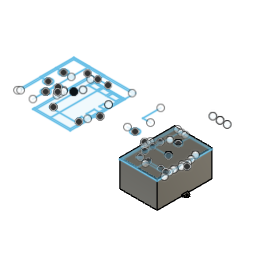
Trab-RICA2 v16 (Autodesk Fusion 360 design; units mm, degrees)
Autodesk Fusion 360 part; units mm, degrees
sketch "Esboço1" plane through (0, 0, 0) normal (0, 0, 1) x (1, 0, 0)
  line L0 (-57.5, 57.5) -> (62.5, 57.5)
  line L1 (62.5, 57.5) -> (62.5, -52.5)
  line L2 (-57.5, -52.5) -> (-57.5, 57.5)
  line L3 (-54.5, -49.5) -> (-54.5, 54.5)
  line L4 (-54.5, 54.5) -> (59.5, 54.5)
  line L5 (-57.5, 57.5) -> (2.5, 57.5)
  line L6 (2.5, 54.5) -> (2.5, 44.5)
  circle A0 centre (2.5, 44.5) radius 3
  line L7 (2.5, 44.5) -> (22.5, 44.5)
  line L8 (2.5, 44.5) -> (-17.5, 44.5)
  circle A1 centre (-17.5, 44.5) radius 3
  circle A2 centre (22.5, 44.5) radius 3
  line L9 (-57.5, 57.5) -> (-27.5, 57.5)
  line L10 (-27.5, 57.5) -> (-27.5, -52.5)
  line L11 (-57.5, 57.5) -> (-57.5, 22.5)
  line L12 (-57.5, 22.5) -> (-42.5, 22.5)
  circle A3 centre (-42.5, 22.5) radius 7.5
  line L13 (-57.5, 22.5) -> (-57.5, -7.5)
  line L14 (-57.5, -7.5) -> (-42.5, -7.5)
  circle A4 centre (-42.5, -7.5) radius 7.5
  line L15 (-27.5, -7.5) -> (-12.5, -7.5)
  circle A5 centre (-27.5, 22.5) radius 3.5
  line L16 (-27.5, -7.5) -> (-27.5, -27.5)
  circle A6 centre (-27.5, -27.5) radius 7.5
  line L17 (-25.25, -25.75) -> (-29.75, -25.75)
  line L18 (-29.75, -25.75) -> (-29.75, -29.25)
  line L19 (-29.75, -29.25) -> (-25.25, -29.25)
  line L20 (-25.25, -29.25) -> (-25.25, -25.75)
  line L21 (-29.4343, -26.0657) -> (-29.4343, -28.9343)
  line L22 (-29.4343, -28.9343) -> (-25.5657, -28.9343)
  line L23 (-25.5657, -28.9343) -> (-25.5657, -26.0657)
  line L24 (-25.5657, -26.0657) -> (-29.4343, -26.0657)
  line L25 (59.5, 35.5) -> (2.5, 35.5)
  line L26 (2.5, 35.5) -> (2.5, -49.5)
  line L27 (59.5, -49.5) -> (56, -49.5)
  line L28 (56, -49.5) -> (56, -46)
  line L29 (2.5, -49.5) -> (6, -49.5)
  line L30 (6, -49.5) -> (6, -46)
  circle A7 centre (6, 12) radius 1.375
  circle A8 centre (6, 12) radius 3
  circle A9 centre (6, -46) radius 1.375
  circle A10 centre (6, -46) radius 3
  circle A11 centre (56, -46) radius 1.375
  circle A12 centre (56, -46) radius 3
  circle A13 centre (56, 12) radius 1.375
  circle A14 centre (56, 12) radius 3
  line L31 (59.5, -49.5) -> (59.5, -38.9)
  line L32 (59.5, -38.9) -> (59.5, -42.9)
  line L33 (59.5, -38.9) -> (59.5, -34.9)
  line L34 (59.5, -42.9) -> (56, -42.9)
  line L35 (59.5, -49.5) -> (59.5, -17.5)
  line L36 (59.5, -17.5) -> (59.5, -25)
  line L37 (59.5, -25) -> (59.5, -32.5)
  line L38 (59.5, -17.5) -> (59.5, -10)
  line L39 (59.5, -49.5) -> (59.5, 4)
  line L40 (59.5, 4) -> (59.5, 0)
  line L41 (59.5, 4) -> (59.5, 8)
  line L42 (59.5, 35.5) -> (49.25, 35.5)
  line L43 (49.25, 35.5) -> (57.25, 35.5)
  line L44 (49.25, 35.5) -> (41.25, 35.5)
  line L45 (41.25, 35.5) -> (41.25, 25)
  line L46 (57.25, 35.5) -> (57.25, 25)
  line L47 (59.5, 35.5) -> (30.5, 35.5)
  line L48 (30.5, 35.5) -> (38, 35.5)
  line L49 (30.5, 35.5) -> (23, 35.5)
  line L50 (38, 35.5) -> (38, 25)
  line L51 (38, 25) -> (23, 25)
  line L52 (41.25, 25) -> (57.25, 25)
  line L53 (59.5, 35.5) -> (12.5, 35.5)
  line L54 (12.5, 35.5) -> (20, 35.5)
  line L55 (12.5, 35.5) -> (5, 35.5)
  line L56 (23, 35.5) -> (23, 25)
  line L57 (20, 35.5) -> (20, 25)
  line L58 (20, 25) -> (5, 25)
  line L59 (5, 25) -> (5, 35.5)
  line L60 (59.5, 8) -> (50, 8)
  line L61 (50, 8) -> (50, 0)
  line L62 (59.5, 0) -> (50, 0)
  line L63 (59.5, -10) -> (50, -10)
  line L64 (50, -10) -> (50, -25)
  line L65 (50, -25) -> (59.5, -25)
  line L66 (59.5, -34.9) -> (50, -34.9)
  line L67 (50, -34.9) -> (50, -42.9)
  line L68 (56, -42.9) -> (50, -42.9)
  line L69 (59.5, 37.5) -> (2.5, 37.5)
  line L70 (2.5, 37.5) -> (-7.5, 37.5)
  line L71 (59.5, 37.5) -> (62.5, 37.5)
  circle A15 centre (-23.226, -7.5) radius 6.5
  line L72 (-7.5, 37.5) -> (-4.5, 37.5)
  line L73 (2.5, 35.5) -> (-7.5, 35.5)
  line L74 (2.5, -49.5) -> (59.5, -49.5)
  line L75 (62.5, -52.5) -> (62.5, -55.5)
  line L76 (59.5, -52.5) -> (59.5, -49.5)
  line L77 (-10.5, -66.5) -> (-10.5, 37.5)
  line L78 (-10.5, 37.5) -> (-7.5, 37.5)
  line L79 (-7.5, -66.5) -> (-7.5, 35.5)
  line L80 (59.5, 35.5) -> (59.5, 8)
  line L81 (21.2759, 35.5) -> (21.2759, -66.5)
  line L82 (21.2759, -66.5) -> (-10.5, -66.5)
  line L83 (-10.5, -66.5) -> (-10.5, -69.5)
  line L84 (-10.5, -69.5) -> (62.5, -69.5)
  line L85 (62.5, -69.5) -> (62.5, -55.5)
  line L86 (21.2759, -66.5) -> (59.5, -66.5)
  line L87 (59.5, -66.5) -> (59.5, -52.5)
  line L88 (62.5, 37.5) -> (62.5, -16)
  line L89 (62.5, -16) -> (67.5, -16)
  circle A16 centre (67.5, -16) radius 1.5
  circle A17 centre (67.5, -16) radius 4
  line L90 (62.5, -22.3696) -> (69.0157, -19.7017)
  line L91 (69.0783, -12.3245) -> (62.5, -9.4998)
  line L92 (-17.0783, -19.675) -> (-10.5, -22.4998)
  circle A18 centre (-15.5, -15.9996) radius 1.5
  line L93 (-10.5, -9.6299) -> (-17.0157, -12.2978)
  circle A19 centre (-15.5, -15.9996) radius 4
  line L94 (-10.5, -15.9996) -> (-15.5, -15.9996)
  point P0 (-27.5, -27.5)
  dimension "d1" = 120
  dimension "d2" = 110
  dimension "d4" = 10
  dimension "d5" = 6
  dimension "d6" = 20
  dimension "d7" = 20
  dimension "d8" = 6
  dimension "d9" = 6
  dimension "d10" = 30
  dimension "d11" = 35
  dimension "d12" = 15
  dimension "d13" = 15
  dimension "d14" = 30
  dimension "d15" = 15
  dimension "d16" = 15
  dimension "d19" = 15
  dimension "d20" = 7
  dimension "d22" = 20
  dimension "d23" = 15
  dimension "d24" = 4.5
  dimension "d25" = 3.5
  dimension "d26" = -0.3157
  dimension "d57" = 57
  dimension "d58" = 57
  dimension "d59" = 3.5
  dimension "d60" = 3.5
  dimension "d61" = 3.5
  dimension "d62" = 3.5
  dimension "d63" = 58
  dimension "d64" = 58
  dimension "d65" = 2.75
  dimension "d66" = 6
  dimension "d67" = 2.75
  dimension "d68" = 6
  dimension "d69" = 2.75
  dimension "d70" = 6
  dimension "d71" = 2.75
  dimension "d72" = 6
  dimension "d73" = 10.6
  dimension "d74" = 4
  dimension "d75" = 4
  dimension "d76" = 32
  dimension "d77" = 7.5
  dimension "d79" = 7.5
  dimension "d80" = 53.5
  dimension "d81" = 4
  dimension "d82" = 4
  dimension "d83" = 10.25
  dimension "d84" = 8
  dimension "d85" = 8
  dimension "d86" = 29
  dimension "d87" = 7.5
  dimension "d88" = 7.5
  dimension "d89" = 47
  dimension "d90" = 7.5
  dimension "d91" = 7.5
  dimension "d92" = 2
  dimension "d94" = 13
  dimension "d95" = 3
  dimension "d118" = 3
  dimension "d131" = 102
  dimension "d132" = 3
  dimension "d242" = 53.5
  dimension "d243" = 5
  dimension "d244" = 3
  dimension "d245" = 8
  dimension "d246" = 5
  dimension "d247" = 3
  dimension "d248" = 8
  constraint horizontal L0
  constraint perpendicular L0 L1
  constraint parallel L1 L2
  constraint midpoint L0 L5.end
  constraint midpoint L4 L6.start
  constraint perpendicular L4 L6
  constraint coincident L6.end A0.centre
  constraint perpendicular L6 L7
  constraint coincident L8.end A1.centre
  constraint coincident L7.end A2.centre
  constraint perpendicular L2 L9
  constraint perpendicular L9 L11
  constraint perpendicular L3 L12
  constraint coincident L12.end A3.centre
  constraint perpendicular L12 L13
  constraint perpendicular L13 L14
  constraint coincident L14.end A4.centre
  constraint coincident L10 L15.start
  constraint perpendicular L10 L15
  constraint perpendicular L15 L16
  constraint coincident P0 L16.end
  constraint horizontal L17
  constraint perpendicular L17 L18
  constraint parallel L17 L19
  constraint parallel L18 L20
  constraint perpendicular L26 L29
  constraint perpendicular L29 L30
  constraint concentric A7 A8
  constraint coincident L30.end A9.centre
  constraint concentric A9 A10
  constraint coincident L28.end A11.centre
  constraint concentric A13 A14
  constraint perpendicular L27 L31
  constraint parallel L31 L32
  constraint perpendicular L27 L35
  constraint parallel L35 L36
  constraint parallel L35 L37
  constraint parallel L39 L40
  constraint parallel L42 L43
  constraint parallel L25 L44
  constraint perpendicular L25 L45
  constraint perpendicular L43 L46
  constraint parallel L25 L47
  constraint parallel L47 L48
  constraint parallel L25 L49
  constraint perpendicular L25 L50
  constraint perpendicular L50 L51
  constraint perpendicular L46 L52
  constraint parallel L25 L53
  constraint parallel L25 L54
  constraint parallel L25 L55
  constraint perpendicular L51 L56
  constraint perpendicular L53 L57
  constraint perpendicular L57 L58
  constraint perpendicular L25 L59
  constraint perpendicular L41 L60
  constraint perpendicular L60 L61
  constraint perpendicular L61 L62
  constraint perpendicular L39 L63
  constraint perpendicular L63 L64
  constraint perpendicular L39 L66
  constraint perpendicular L34 L67
  constraint perpendicular L67 L68
  constraint coincident L1 L71.end
  constraint perpendicular L1 L71
  constraint coincident L15 A15.centre
  constraint perpendicular L26 L74
  constraint parallel L1 L75
  constraint perpendicular L27 L76
  constraint perpendicular L73 L79
  constraint perpendicular L60 L80
  constraint coincident L25 L81.start
  constraint coincident L79.start L82
  constraint perpendicular L79 L82
  constraint perpendicular L77 L82
  constraint perpendicular L82 L83
  constraint perpendicular L75 L84
  constraint perpendicular L84 L85
  constraint perpendicular L76 L86
  constraint perpendicular L71 L88
  constraint perpendicular L1 L89
  constraint coincident L89.end A16.centre
  constraint concentric A16 A17
  constraint coincident L1 L90.start
  constraint coincident A17 L90.end
  constraint tangent A17 L90
  constraint coincident A17 L91.start
  constraint coincident L1 L91.end
  constraint tangent A17 L91
  constraint coincident A18.centre A19.centre
  constraint concentric A18 A19
  constraint coincident L93.end A19
  constraint tangent L93 A19
  constraint coincident L92.start A19
  constraint tangent L92 A19
  measures "d1" distance of L1.end L2.start
  measures "d2" distance of L0.end L1.end
  measures "d4" distance of L6.start L6.end
  measures "d5" diameter of A0
  measures "d6" distance of L6.end L7.end
  measures "d7" distance of L6.end L8.end
  measures "d8" diameter of A1
  measures "d9" diameter of A2
  measures "d10" distance of L0.start L9.end
  measures "d11" distance of L0.start L11.end
  measures "d12" distance of L11.end L12.end
  measures "d13" diameter of A3
  measures "d14" distance of L11.end L13.end
  measures "d15" distance of L13.end L14.end
  measures "d16" diameter of A4
  measures "d19" distance of L15.start L15.end
  measures "d20" diameter of A5
  measures "d22" distance of L15.start P0
  measures "d23" diameter of A6
  measures "d24" distance of L18.end L19.end
  measures "d25" distance of L17.end L18.end
  measures "d57" distance of L27.start L26.end
  measures "d58" distance of L25.start L25.end
  measures "d59" distance of L27.start L27.end
  measures "d60" distance of L27.end L28.end
  measures "d61" distance of L26.end L29.end
  measures "d62" distance of L29.end L30.end
  measures "d63" distance of L30.end A7.centre
  measures "d64" distance of L28.end A13.centre
  measures "d65" diameter of A7
  measures "d66" diameter of A8
  measures "d67" diameter of A9
  measures "d68" diameter of A10
  measures "d69" diameter of A11
  measures "d70" diameter of A12
  measures "d71" diameter of A13
  measures "d72" diameter of A14
  measures "d73" distance of L27.start L31.end
  measures "d74" distance of L31.end L32.end
  measures "d75" distance of L31.end L33.end
  measures "d76" distance of L27.start L35.end
  measures "d77" distance of L35.end L36.end
  measures "d79" distance of L35.end L38.end
  measures "d80" distance of L27.start L39.end
  measures "d81" distance of L39.end L40.end
  measures "d82" distance of L39.end L41.end
  measures "d83" distance of L25.start L42.end
  measures "d84" distance of L42.end L43.end
  measures "d85" distance of L42.end L44.end
  measures "d86" distance of L25.start L47.end
  measures "d87" distance of L47.end L48.end
  measures "d88" distance of L47.end L49.end
  measures "d89" distance of L25.start L53.end
  measures "d90" distance of L53.end L54.end
  measures "d91" distance of L53.end L55.end
  measures "d94" diameter of A15
  measures "d95" distance of L70.end L72.end
  measures "d118" distance of L1.end L75.end
  measures "d131" distance of L81.start L81.end
  measures "d132" distance of L77.start L83.end
  measures "d242" distance of L71.end L88.end
  measures "d243" distance of L88.end L89.end
  measures "d244" diameter of A16
  measures "d245" diameter of A17
  measures "d246" distance of L94.start A18.centre
  measures "d247" diameter of A18
  measures "d248" diameter of A19
sketch "Esboço2" plane through (0, 0, 0) normal (0, 0, 1) x (1, 0, 0)
  line L0 (121.4343, 17.9343) -> (117.5657, 17.9343)
  circle A0 centre (119.5, 16.5) radius 7.5
  line L1 (92.5, 57.5) -> (152.5, 57.5)
  circle A1 centre (121.5, 44.5) radius 3
  line L2 (209.5, 54.5) -> (209.5, -49.5)
  line L3 (117.5657, 17.9343) -> (117.5657, 15.0657)
  line L4 (121.4343, 15.0657) -> (121.4343, 17.9343)
  circle A2 centre (113.3812, 29.2702) radius 3.5
  line L5 (212.5, 57.5) -> (212.5, -52.5)
  line L6 (121.5, 44.5) -> (107.5, 44.5)
  line L7 (92.5, 57.5) -> (122.5, 57.5)
  line L8 (98.3812, 29.2702) -> (113.3812, 29.2702)
  line L9 (209.5, -49.5) -> (95.5, -49.5)
  line L10 (92.5, -7.5) -> (107.5, -7.5)
  line L11 (121.75, 14.75) -> (121.75, 18.25)
  line L12 (121.5, 44.5) -> (135.5, 44.5)
  line L13 (121.75, 18.25) -> (117.25, 18.25)
  circle A3 centre (107.5, 44.5) radius 3
  line L14 (117.25, 14.75) -> (121.75, 14.75)
  circle A4 centre (127.764, 29.9834) radius 5
  line L15 (92.5, 22.5) -> (107.5, 22.5)
  line L16 (95.5, 54.5) -> (209.5, 54.5)
  line L17 (92.5, -52.5) -> (92.5, 57.5)
  line L18 (117.5657, 15.0657) -> (121.4343, 15.0657)
  line L19 (95.5, -49.5) -> (95.5, 54.5)
  line L20 (212.5, -52.5) -> (92.5, -52.5)
  line L21 (92.5, 57.5) -> (212.5, 57.5)
  circle A5 centre (135.5, 44.5) radius 3
  line L22 (117.25, 18.25) -> (117.25, 14.75)
  line L23 (92.5, 57.5) -> (92.5, 22.5)
  line L24 (92.5, 22.5) -> (92.5, -7.5)
  line L25 (95.5, 6.594) -> (145, 6.594)
  line L26 (145, 6.594) -> (145, 54.5)
  point P0 (150, 0)
  point P1 (150, 0)
  point P2 (119.5, 16.5)
  dimension "d29" = 3
  dimension "d30" = -0.3157
  dimension "d31" = 120
  dimension "d32" = 110
  dimension "d34" = 6
  dimension "d37" = 6
  dimension "d38" = 6
  dimension "d39" = 30
  dimension "d40" = 35
  dimension "d43" = 30
  dimension "d46" = 15
  dimension "d48" = 7
  dimension "d49" = 10
  dimension "d51" = 15
  dimension "d52" = 4.5
  dimension "d53" = 3.5
  constraint horizontal L21
  constraint perpendicular L5 L21
  constraint parallel L20 L21
  constraint parallel L5 L17
  constraint coincident P1 P0
  constraint midpoint L1.end L21
  constraint coincident A1.centre L6.start
  constraint coincident L6.end A3.centre
  constraint coincident L12.end A5.centre
  constraint perpendicular L7 L17
  constraint perpendicular L7 L23
  constraint perpendicular L15 L19
  constraint perpendicular L15 L24
  constraint perpendicular L10 L24
  constraint coincident A2.centre L8.end
  constraint horizontal L13
  constraint perpendicular L13 L22
  constraint parallel L13 L14
  constraint parallel L11 L22
  constraint coincident L19 L25.start
  constraint perpendicular L19 L25
  constraint coincident L16 L26.end
  constraint perpendicular L16 L26
  measures "d31" distance of L17.start L5.end
  measures "d32" distance of L5.start L5.end
  measures "d34" diameter of A1
  measures "d37" diameter of A3
  measures "d38" diameter of A5
  measures "d39" distance of L1.start L7.end
  measures "d40" distance of L1.start L15.start
  measures "d43" distance of L15.start L10.start
  measures "d46" distance of L8.start A2.centre
  measures "d48" diameter of A2
  measures "d49" diameter of A4
  measures "d51" diameter of A0
  measures "d52" distance of L11.start L14.start
  measures "d53" distance of L13.end L14.start
extrude "Extrusão2" add sketch "Esboço2" along normal blind 3 contours A0 | L16 L19 L25 L26 | L11 L13 L14 L22 makes body 1
extrude "Extrusão3" add sketch "Esboço1" along normal blind 30 separate body contours L1 L69 L70 L71 L72 L75 L77 L78 L83 L84 L85 L88 makes body 2
extrude "Extrusão4" add sketch "Esboço1" along normal blind 3 contours L25 L27 L31 L34 L35 L37 L39 L42 L45 L46 L47 L50 L51 L52 L53 L56 L60 L61 L62 L63 L64 L65 L66 L67 L68 L74 L80 L81 | L25 L42 L43 L44 L45 L46 L47 L52 L53 | L39 L40 L41 L60 L61 L62 | L25 L47 L48 L49 L50 L51 L53 L56 | L35 L36 L38 L39 L63 L64 L65 | L25 L26 L29 L53 L57 L58 L59 L74 L81 | L25 L53 L54 L55 L57 L58 L59 | L26 L29 L73 L74 L79 L81 L82 | L27 L74 L76 L81 L86 L87 | L31 L32 L33 L34 L35 L39 L66 L67 L68 | A7 | A8 | A13 | A14 bodies 2
extrude "Extrusão6" add sketch "Esboço1" along normal blind 8 contours A8 | A10 | A12 | A14 bodies 2
sketch "Esboço3" plane through (0, 37.5, 0) normal (0, 1, 0) x (-1, 0, 0)
  line L0 (-62.5, 0) -> (10.5, 0)
  line L1 (10.5, 30) -> (-62.5, 30)
  line L2 (-62.5, 30) -> (-62.5, 0)
  line L3 (-59.5623, 0) -> (-59.5623, 8)
  line L4 (-2.4095, 0) -> (-2.4095, 8)
  line L5 (-59.5623, 8) -> (-2.4095, 8)
  line L6 (-59.5623, 8) -> (-59.5623, 23)
  line L7 (-2.4095, 8) -> (-2.4095, 23)
  line L8 (-59.5623, 23) -> (-2.4095, 23)
  line L9 (10.5, 0) -> (10.5, 30)
  dimension "d104" = 8
  dimension "d105" = 8
  dimension "d106" = 15
  dimension "d107" = 15
  constraint coincident L0 L3.start
  constraint perpendicular L0 L3
  constraint coincident L0 L4.start
  constraint perpendicular L0 L4
  constraint perpendicular L5 L6
  constraint perpendicular L5 L7
  constraint perpendicular L7 L8
  measures "d104" distance of L3.start L3.end
  measures "d105" distance of L4.start L4.end
  measures "d106" distance of L3.end L6.end
  measures "d107" distance of L4.end L7.end
extrude "Extrusão7" cut sketch "Esboço3" against normal blind 5 contours L5 L6 L7 L8 bodies 2
sketch "Esboço4" plane through (62.5, 0, 0) normal (1, 0, 0) x (0, 1, 0)
  line L0 (-69.5, 0) -> (37.5, 0)
  line L1 (37.5, 0) -> (37.5, 30)
  line L2 (37.5, 30) -> (-69.5, 30)
  line L3 (-43.5, 0) -> (-43.5, 8)
  line L4 (9, 0) -> (9, 8)
  line L5 (-43.5, 8) -> (9, 8)
  line L6 (-43.5, 8) -> (-43.5, 16)
  line L7 (-43.5, 16) -> (9, 16)
  line L8 (9, 16) -> (9, 8)
  line L9 (-69.5, 30) -> (-69.5, 0)
  dimension "d111" = 8
  dimension "d112" = 8
  dimension "d113" = 8
  constraint coincident L0 L3.start
  constraint perpendicular L0 L3
  constraint coincident L0 L4.start
  constraint perpendicular L0 L4
  constraint perpendicular L4 L5
  constraint perpendicular L5 L6
  constraint perpendicular L4 L7
  constraint perpendicular L5 L8
  measures "d111" distance of L3.start L3.end
  measures "d112" distance of L4.start L4.end
  measures "d113" distance of L3.end L6.end
extrude "Extrusão8" cut sketch "Esboço4" against normal blind 5 contours L5 L6 L7 L8 bodies 2
sketch "Esboço5" plane through (0, 0, 3) normal (0, 0, 1) x (-1, 0, 0)
  line L0 (-59.5, -35.5) -> (7.5, -35.5)
  line L1 (-1.5, 53.5) -> (-1.5, 65.5)
  line L2 (7.5, -35.5) -> (7.5, -34.5)
  line L3 (7.5, -34.5) -> (-1.5, -34.5)
  line L4 (-1.5, -34.5) -> (-1.5, -22.5)
  line L5 (7.5, -22.5) -> (7.5, -34.5)
  line L6 (7.5, -35.5) -> (7.5, 66.5)
  line L7 (-1.5, 53.5) -> (7.5, 53.5)
  line L8 (-1.5, 65.5) -> (7.5, 65.5)
  line L9 (7.5, 65.5) -> (7.5, 53.5)
  line L10 (7.5, -22.5) -> (-1.5, -22.5)
  line L11 (7.5, 65.5) -> (4.5, 65.5)
  line L12 (4.5, 65.5) -> (4.5, -34.5)
  line L13 (7.5, -34.5) -> (7.5, 65.5)
  line L14 (7.5, 66.5) -> (-59.5, 66.5)
  circle A0 centre (-56, -12) radius 3
  line L15 (-59.5, 66.5) -> (-59.5, -35.5)
  circle A1 centre (-56, 46) radius 3
  circle A2 centre (-6, 46) radius 3
  circle A3 centre (-6, -12) radius 3
  line L16 (-56.5, 53.5) -> (-47.5, 53.5)
  line L17 (-47.5, 65.5) -> (-50.5, 65.5)
  line L18 (-56.5, 65.5) -> (-47.5, 65.5)
  line L19 (-56.5, 53.5) -> (-56.5, 65.5)
  line L20 (-47.5, 65.5) -> (-47.5, 53.5)
  line L21 (-56.5, 65.5) -> (-53.5, 65.5)
  line L22 (-53.5, 65.5) -> (-53.5, 53.5)
  line L23 (4.5, -22.5) -> (-1.5, -34.5)
  line L24 (-1.5, -22.5) -> (4.5, -34.5)
  circle A4 centre (1.5, -28.5) radius 1.25
  line L25 (-1.5, 53.5) -> (4.5, 65.5)
  line L26 (4.5, 53.5) -> (-1.5, 65.5)
  circle A5 centre (1.5, 59.5) radius 1.25
  line L27 (-53.5, 53.5) -> (-47.5, 65.5)
  line L28 (-47.5, 53.5) -> (-53.5, 65.5)
  circle A6 centre (-50.5, 59.5) radius 1.25
  dimension "d117" = 12
  dimension "d120" = 1
  dimension "d121" = 9
  dimension "d122" = 12
  dimension "d126" = 9
  dimension "d127" = 9
  dimension "d128" = 3
  dimension "d133" = 12
  dimension "d134" = 9
  dimension "d135" = 9
  dimension "d137" = 3
  dimension "d148" = 2.5
  dimension "d232" = 2.5
  dimension "d233" = 2.5
  constraint coincident L0.end L2.start
  constraint perpendicular L0 L2
  constraint perpendicular L3 L4
  constraint perpendicular L1 L7
  constraint perpendicular L6 L8
  constraint perpendicular L7 L9
  constraint perpendicular L4 L10
  constraint perpendicular L6 L11
  constraint coincident L3 L12.end
  constraint perpendicular L3 L12
  constraint perpendicular L8 L13
  constraint perpendicular L16 L19
  constraint perpendicular L16 L20
  constraint perpendicular L19 L21
  constraint coincident L16 L22.end
  constraint perpendicular L16 L22
  constraint coincident L12 L23.start
  constraint coincident L10 L23.start
  constraint midpoint L24 A4.centre
  constraint coincident L7 L26.start
  constraint coincident L12 L26.start
  constraint midpoint L25 A5.centre
  constraint midpoint L27 A6.centre
  measures "d117" distance of L1.start L1.end
  measures "d120" distance of L0.end L2.end
  measures "d121" distance of L2.end L3.end
  measures "d122" distance of L3.end L4.end
  measures "d126" distance of L1.start L7.end
  measures "d127" distance of L1.end L8.end
  measures "d128" distance of L8.end L11.end
  measures "d133" distance of L18.start L16.start
  measures "d134" distance of L16.start L16.end
  measures "d135" distance of L18.start L17.start
  measures "d137" distance of L18.start L21.end
  measures "d148" diameter of A4
  measures "d232" diameter of A5
  measures "d233" diameter of A6
extrude "Extrusão9" add sketch "Esboço5" along normal blind 37 separate body contours L3 L5 L6 L10 L12 L13 | L6 L7 L8 L9 L11 L12 L13 | L16 L18 L19 L21 L22 makes body 3 at (-7.5, -57.5, 27.6667) makes body 4 at (-7.5, 26.5, 15.3333) makes body 5 at (56.5, -57.5, 27.6667)
sketch "Esboço6" plane through (0, 0, 40) normal (0, 0, 1) x (-1, 0, 0)
  line L0 (7.5, 53.5) -> (7.5, 65.5)
  line L1 (7.5, 65.5) -> (4.5, 65.5)
  line L2 (4.5, 65.5) -> (4.5, 53.5)
  line L3 (4.5, -34.5) -> (7.5, -34.5)
  line L4 (7.5, 65.5) -> (-56.5, 65.5)
  line L5 (-56.5, 65.5) -> (-56.5, 53.5)
  line L6 (4.5, 53.5) -> (7.5, 53.5)
  line L7 (7.5, -34.5) -> (7.5, -22.5)
  line L8 (7.5, -22.5) -> (4.5, -22.5)
  line L9 (4.5, -22.5) -> (4.5, -34.5)
  line L10 (7.5, 65.5) -> (7.5, -34.5)
  line L11 (7.5, -34.5) -> (-56.5, -34.5)
  line L12 (-56.5, -34.5) -> (-56.5, 65.5)
  line L13 (4.5, 62.5) -> (-53.5, 62.5)
  line L14 (-53.5, -31.5) -> (-53.5, 62.5)
  line L15 (4.5, -31.5) -> (-53.5, -31.5)
  line L16 (4.5, 62.5) -> (4.5, -31.5)
  dimension "d147" = 3
  constraint coincident L0.end L1.start
  constraint perpendicular L0 L4
  constraint perpendicular L3 L5
  constraint coincident L3.end L7.start
  constraint perpendicular L5 L11
  constraint perpendicular L4 L12
hole "Furo1" at (50.5, -59.5, 3) direction (0, 0, -1) diameter 2.5 depth 2 tip angle 118 bodies 2
hole "Furo2" at (-1.5, 28.5, 3) at (-1.5, -59.5, 3) direction (0, 0, -1) diameter 2.5 depth 2 tip angle 118 bodies 2
extrude "Extrusão11" add sketch "Esboço6" along normal blind 2 contours L0 L1 L2 L4 L6 L10 L16 | L6 L8 L10 L16 | L3 L7 L8 L9 L10 L11 L16 | L2 L4 L5 L9 L11 L12 L13 L14 L15 bodies 2 5 3 4
sketch "Esboço7" plane through (0, 0, 0) normal (0, 0, 1) x (1, 0, 0)
  line L0 (229.5, 35.5) -> (172.5, 35.5)
  line L1 (182.5, 35.5) -> (175, 35.5)
  line L2 (172.5, 35.5) -> (172.5, -49.5)
  line L3 (172.5, 35.5) -> (162.5, 35.5)
  line L4 (172.5, 37.5) -> (162.5, 37.5)
  line L5 (229.5, 37.5) -> (172.5, 37.5)
  line L6 (112.5, 57.5) -> (112.5, 22.5)
  line L7 (112.5, 22.5) -> (127.5, 22.5)
  line L8 (112.5, -7.5) -> (127.5, -7.5)
  circle A0 centre (127.5, -7.5) radius 7.5
  line L9 (159.5, -66.5) -> (159.5, 37.5)
  line L10 (162.5, -66.5) -> (162.5, 35.5)
  line L11 (159.5, -69.5) -> (232.5, -69.5)
  line L12 (172.5, -49.5) -> (229.5, -49.5)
  line L13 (229.5, 4) -> (229.5, 0)
  line L14 (229.5, -49.5) -> (229.5, 4)
  line L15 (229.5, 35.5) -> (229.5, 8)
  circle A1 centre (226, 12) radius 3
  circle A2 centre (226, 12) radius 1.375
  line L16 (229.5, 4) -> (229.5, 8)
  circle A3 centre (226, -46) radius 3
  circle A4 centre (226, -46) radius 1.375
  line L17 (229.5, -49.5) -> (226, -49.5)
  line L18 (226, -49.5) -> (226, -46)
  line L19 (229.5, -52.5) -> (229.5, -49.5)
  line L20 (229.5, -66.5) -> (229.5, -52.5)
  line L21 (229.5, -49.5) -> (229.5, -38.9)
  line L22 (229.5, -49.5) -> (229.5, -17.5)
  circle A5 centre (176, 12) radius 3
  circle A6 centre (176, 12) radius 1.375
  circle A7 centre (176, -46) radius 3
  circle A8 centre (176, -46) radius 1.375
  line L23 (176, -49.5) -> (176, -46)
  line L24 (172.5, -49.5) -> (176, -49.5)
  line L25 (229.5, -38.9) -> (229.5, -42.9)
  line L26 (229.5, -38.9) -> (229.5, -34.9)
  line L27 (159.5, -69.5) -> (159.5, -66.5)
  line L28 (162.5, -66.5) -> (229.5, -66.5)
  line L29 (232.5, -52.5) -> (232.5, -69.5)
  line L30 (159.5, 37.5) -> (162.5, 37.5)
  line L31 (229.5, 37.5) -> (232.5, 37.5)
  line L32 (232.5, -52.5) -> (232.5, 37.5)
  line L33 (159.5, -69.5) -> (159.5, -16)
  line L34 (159.5, -16) -> (170, -16)
  circle A9 centre (205.5, 94.5) radius 3
  circle A10 centre (191.5, 94.5) radius 3
  circle A11 centre (177.5, 94.5) radius 3
  circle A12 centre (191.5, 94.5) radius 3
  circle A13 centre (205.5, 94.5) radius 3
  circle A14 centre (177.5, 94.5) radius 3
  circle A15 centre (191.5, 94.5) radius 3
  circle A16 centre (170, -16) radius 3.25
  line L35 (170, -16) -> (170, -31)
  circle A17 centre (170, -31) radius 3.25
  line L36 (170, -16) -> (170, -1)
  circle A18 centre (170, -1) radius 3.25
  line L37 (162.5, -66.5) -> (190.5, -66.5)
  line L38 (190.5, -66.5) -> (190.5, -45)
  line L39 (190.5, 35.5) -> (190.5, 14)
  circle A19 centre (190.5, -45) radius 3.5
  circle A20 centre (190.5, 14) radius 6
  line L40 (173.25, -16.0046) -> (201.25, -16.0046)
  line L41 (190.5, -45) -> (215.5, -45)
  circle A21 centre (215.5, -45) radius 5
  line L42 (199.5, -13.7546) -> (203, -13.7546)
  line L43 (203, -13.7546) -> (203, -18.2546)
  line L44 (203, -18.2546) -> (199.5, -18.2546)
  line L45 (199.5, -18.2546) -> (199.5, -13.7546)
  line L46 (199.5, -13.7546) -> (203, -18.2546) construction
  line L47 (203, -13.7546) -> (199.5, -18.2546) construction
  line L48 (199.81, -17.9446) -> (199.81, -14.0646)
  line L49 (199.81, -14.0646) -> (202.69, -14.0646)
  line L50 (202.69, -14.0646) -> (202.69, -17.9446)
  line L51 (202.69, -17.9446) -> (199.81, -17.9446)
  circle A22 centre (201.25, -16.0046) radius 5
  line L52 (239.0783, -12.3245) -> (232.5, -9.4998)
  circle A23 centre (237.5, -16) radius 1.5
  line L53 (232.5, -22.3696) -> (239.0157, -19.7017)
  circle A24 centre (237.5, -16) radius 4
  line L54 (232.5, -16) -> (237.5, -16)
  line L55 (152.9217, -19.675) -> (159.5, -22.4998)
  circle A25 centre (154.5, -15.9996) radius 1.5
  line L56 (159.5, -9.6299) -> (152.9843, -12.2978)
  circle A26 centre (154.5, -15.9996) radius 4
  line L57 (159.5, -15.9996) -> (154.5, -15.9996)
  point P0 (165.5, 37.5)
  point P1 (229.5, -32.5)
  point P2 (170, 0)
  point P3 (232.5, -55.5)
  point P4 (191.6698, -51.602)
  point P5 (201.25, -16.0046)
  dimension "d149" = 2
  dimension "d155" = 35
  dimension "d156" = 15
  dimension "d158" = 30
  dimension "d159" = 15
  dimension "d160" = 15
  dimension "d194" = 3
  dimension "d195" = 53.5
  dimension "d197" = 6
  dimension "d198" = 6
  dimension "d199" = 6
  dimension "d205" = 6
  dimension "d206" = 6
  dimension "d207" = 6
  dimension "d208" = 6
  dimension "d209" = 6.5
  dimension "d210" = 15
  dimension "d211" = 6.5
  dimension "d212" = 15
  dimension "d213" = 6.5
  dimension "d215" = 28
  dimension "d216" = 21.5
  dimension "d217" = 21.5
  dimension "d218" = 7
  dimension "d219" = 12
  dimension "d220" = 25
  dimension "d221" = 10
  dimension "d222" = 3.5
  dimension "d223" = 4.5
  dimension "d224" = 0.31
  dimension "d225" = 10
  dimension "d252" = 5
  dimension "d253" = 3
  dimension "d254" = 8
  dimension "d255" = 5
  dimension "d256" = 3
  dimension "d257" = 8
  constraint coincident L8.end A0.centre
  constraint perpendicular L2 L24
  constraint perpendicular L23 L24
  constraint concentric A5 A6
  constraint coincident A7.centre A8.centre
  constraint concentric A7 A8
  constraint coincident A3.centre A4.centre
  constraint concentric A1 A2
  constraint perpendicular L17 L21
  constraint parallel L21 L25
  constraint perpendicular L17 L22
  constraint parallel L13 L14
  constraint parallel L0 L1
  constraint perpendicular L2 L12
  constraint perpendicular L17 L19
  constraint perpendicular L3 L10
  constraint perpendicular L11 L27
  constraint perpendicular L20 L28
  constraint perpendicular L11 L29
  constraint perpendicular L9 L30
  constraint perpendicular L31 L32
  constraint perpendicular L11 L33
  constraint perpendicular L10 L34
  constraint coincident L34.end A16.centre
  constraint perpendicular L34 L35
  constraint coincident L35.end A17.centre
  constraint perpendicular L34 L36
  constraint coincident L36.end A18.centre
  constraint coincident A16 L40.start
  constraint perpendicular L10 L37
  constraint coincident L0 L39.start
  constraint perpendicular L37 L38
  constraint perpendicular L0 L39
  constraint coincident L38.end A19.centre
  constraint coincident L39.end A20.centre
  constraint perpendicular L2 L40
  constraint perpendicular L38 L41
  constraint coincident L41.end A21.centre
  constraint horizontal L42
  constraint perpendicular L42 L43
  constraint parallel L42 L44
  constraint parallel L43 L45
  constraint coincident L46 P5
  constraint coincident L47 P5
  constraint coincident P5 L40.end
  constraint coincident A23.centre A24.centre
  constraint concentric A23 A24
  constraint coincident L53.end A24
  constraint tangent L53 A24
  constraint coincident L52.start A24
  constraint tangent L52 A24
  constraint coincident A25.centre A26.centre
  constraint concentric A25 A26
  constraint coincident L56.end A26
  constraint tangent L56 A26
  constraint coincident L55.start A26
  constraint tangent L55 A26
  measures "d155" distance of L6.start L6.end
  measures "d156" distance of L6.end L7.end
  measures "d158" distance of L6.end L8.start
  measures "d159" distance of L8.start L8.end
  measures "d160" diameter of A0
  measures "d194" distance of L9.start L11.start
  measures "d195" distance of L11.start L33.end
  measures "d197" diameter of A10
  measures "d198" diameter of A11
  measures "d199" diameter of A9
  measures "d205" diameter of A12
  measures "d206" diameter of A14
  measures "d207" diameter of A13
  measures "d208" diameter of A15
  measures "d209" diameter of A16
  measures "d210" distance of L34.end L35.end
  measures "d211" diameter of A17
  measures "d212" distance of L34.end L36.end
  measures "d213" diameter of A18
  measures "d215" distance of L10.start L37.end
  measures "d216" distance of L39.start L39.end
  measures "d217" distance of L37.end L38.end
  measures "d218" diameter of A19
  measures "d219" diameter of A20
  measures "d220" distance of L38.end L41.end
  measures "d221" diameter of A21
  measures "d222" distance of L43.end L44.end
  measures "d223" distance of L42.end L43.end
  measures "d225" diameter of A22
  measures "d252" distance of L54.start A23.centre
  measures "d253" diameter of A23
  measures "d254" diameter of A24
  measures "d255" distance of L57.start A25.centre
  measures "d256" diameter of A25
  measures "d257" diameter of A26
extrude "Extrusão13" add sketch "Esboço7" along normal blind 3 separate body contours L0 L1 L2 L12 L13 L14 L15 L16 L17 L21 L22 L24 L25 L26 A16 A17 A18 L38 A19 L41 A21 | L2 L3 L10 L34 A16 L36 A18 | L2 A16 L36 A18 | L2 L10 L12 L24 L28 L34 A16 L35 A17 L37 L38 | L2 A16 L35 A17 | L12 L17 L19 L20 L28 L38 A21 | L12 L38 A19 L41 A21 | L12 A21 | L12 A21 | L4 L5 L9 L11 L27 L29 L30 L31 L32 L33 | A1 | A2 | A3 | A4 | A5 | A6 | A7 | A8 makes body 6
extrude "Extrusão14" add sketch "Esboço7" against normal blind 50 contours L4 L5 L9 L11 L27 L29 L30 L31 L32 L33 bodies 6
extrude "Extrusão16" add sketch "Esboço5" along normal blind 5 contours L12 L23 L24 A4 | L3 L23 L24 A4 | L4 L23 L24 A4 | L10 L23 L24 A4 | L8 L25 L26 A5 | L12 L25 L26 A5 | L7 L25 L26 A5 | L1 L25 L26 A5 | L16 L27 L28 A6 | L22 L27 L28 A6 | L20 L27 L28 A6 | L17 L18 L27 L28 A6 bodies 5
extrude "Extrusão15" add sketch "Esboço1" along normal blind 3 contours A9 | A11 bodies 2 5
extrude "Extrusão17" add sketch "Esboço1" against normal blind 2.5 from surface at 30 contours L1 L88 L89 A17 L91 | L1 L89 A17 L90 | A17 | L77 L93 A19 L94 | L77 L92 A19 L94 | A19 bodies 2
extrude "Extrusão18" add sketch "Esboço7" along normal blind 2.5 from surface at -50 contours L9 L56 A26 L57 | L32 L52 A24 L54 | L9 L33 L55 A26 L57 | A26 | L32 L53 A24 L54 | A24 bodies 6
extrude "Extrusão19" add sketch "Esboço7" along normal blind 4 contours A22 bodies 6
extrude "Extrusão20" add sketch "Esboço7" along normal blind 5 contours L42 L43 L44 L45 bodies 6
hidden bodies 1 2 5
named bodies: "Teste Buracos", "Base Case", "Tamp Case", "Suporte PCB"
